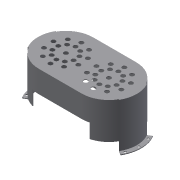
# Autodesk Inventor part: Gear Cover
Saved by Autodesk Inventor 2016 (Build 200138000, 138)
## iProperties
Created: 2012-10-11
Part Number: Gear Cover
Material: Generic
Document SubType Name: Sheet Metal
Designer: bruno.silveira
Density: 1 g/cm^3
Sheet Metal Rule: Default_mm
Flat Pattern Width: 75 cm
Flat Pattern Length: 33.7048 cm
Flat Pattern Area: 2527.86 cm^2
Sheet Metal Width: 750.000 mm
Sheet Metal Length: 337.048 mm
Sheet Metal Area: 252785.840 mm^2
Appearance: Default
Mass: 3205.56 g
Surface Area: 13697.7 cm^2
Volume: 3205.56 cm^3
Author: bruno.silveira
Autodesk Inventor part; units mm, degrees
ref_plane "YZ Plane" through (0, 0, 0) normal (1, 0, 0) x (0, 1, 0)
ref_plane "XZ Plane" through (0, 0, 0) normal (0, 1, 0) x (-1, 0, 0)
ref_plane "XY Plane" through (0, 0, 0) normal (0, 0, 1) x (1, 0, 0)
sketch "Sketch1" plane through (0, 0, 0) normal (0, 0, 1) x (1, 0, 0)
  circle A0 centre (0, 0) radius 190
  circle A1 centre (300, 0) radius 190
  line L0 (0, 190) -> (300, 190)
  line L1 (0, -190) -> (300, -190)
  dimension "d0" = 380
  dimension "d1" = 380
  dimension "d2" = 300
  measures "d0" diameter of A0
  measures "d1" diameter of A1
  measures "d2" distance of point (0, 0) A1.centre
extrude "Plate1" add sketch "Sketch1" along normal blind 4
sketch "Sketch2" plane through (0, 0, 0) normal (0, 0, -1) x (-1, 0, 0)
  arc A0 (-300, 190) -> (-300, -190) centre (-300, 0) ccw projected
  line L0 (0, -190) -> (-300, -190) projected
  arc A1 (0, -190) -> (0, 190) centre (0, 0) ccw projected
  line L1 (-300, 190) -> (0, 190) projected
  arc A2 (0, -186) -> (0, 186) centre (0, 0) ccw
  line L2 (0, -186) -> (-300, -186)
  arc A3 (-300, 186) -> (-300, -186) centre (-300, 0) ccw
  line L3 (-300, 186) -> (0, 186)
  dimension "d4" = 4
  constraints: 4 end point, 4 point on circle, 2 centre point, 3 other
  measures "d4" distance between parallel lines of L1 L3
extrude "Extrusion1" add sketch "Sketch2" along normal blind 250
sketch "Sketch3" plane through (0, 0, 4) normal (0, 0, 1) x (1, 0, 0)
  arc A0 (300, -190) -> (300, 190) centre (300, 0) ccw projected
  arc A1 (0, 190) -> (0, -190) centre (0, 0) ccw projected
  circle A2 centre (0, 0) radius 15
  circle A3 centre (300, 0) radius 15
  circle A4 centre (300, 0) radius 117.5
  circle A5 centre (408.5558, 44.9653) radius 15
  circle A6 centre (300, 0) radius 72.5
  circle A7 centre (366.9813, 27.7445) radius 15
  circle A8 centre (0, 0) radius 117.5
  circle A9 centre (0, 0) radius 72.5
  circle A10 centre (117.5, 0) radius 15
  circle A11 centre (72.5, 0) radius 15
  dimension "d29" = 235
  dimension "d30" = 145
  dimension "d7" = 30
  dimension "d8" = 30
  dimension "d11" = 235
  dimension "d12" = 30
  dimension "d13" = 145
  dimension "d14" = 30
  dimension "d31" = 30
  dimension "d32" = 30
  constraints: 8 centre point, 5 coincident, 2 horizontal alignment, 4 other
  measures "d7" diameter of A2
  measures "d8" diameter of A3
  measures "d11" diameter of A4
  measures "d12" diameter of A5
  measures "d13" diameter of A6
  measures "d14" diameter of A7
  measures "d31" diameter of A10
  measures "d32" diameter of A11
hole "Hole2" at (408.5558, 44.9653, 4) at (366.9813, 27.7445, 4) at (300, 0, 4) direction (0, 0, -1) diameter 30 depth 4 tip angle 118
pattern_circular "Circular Pattern2" count 10 over 360 about axis through (300, 0, 2) along (0, 0, 1) of "Hole2"
pattern_linear "Rectangular Pattern2" count 2 spacing 300 along (-1, 0, 0) of "Hole2", "Circular Pattern2"
sketch "Sketch4" plane through (0, -190, 4) normal (0, -1, 0) x (1, 0, 0)
  line L0 (0, -254) -> (0, 0) projected
  line L1 (0, -254) -> (300, -254) projected
  line L2 (-50, -154) -> (350, -154)
  line L3 (350, -154) -> (350, -254)
  line L4 (350, -254) -> (-50, -254)
  line L5 (-50, -254) -> (-50, -154)
  point P0 (0, -4)
  dimension "d49" = 400
  dimension "d50" = 50
  dimension "d51" = 100
  dimension "d52" = 0
  constraints: 8 end point, 2 parallel, 1 horizontal, 1 perpendicular
  measures "d49" distance of L3.end L4.end
  measures "d50" distance between parallel lines of L0 L5
  measures "d51" distance of L2.end L3.end
  measures "d52" distance between parallel lines of L1 L4
extrude "Cut1" cut sketch "Sketch4" against normal blind 10
sketch "Sketch5" plane through (0, 0, -250) normal (0, 0, -1) x (-1, 0, 0)
  line L0 (-300, 186) -> (0, 186) projected
  line L1 (-300, 190) -> (0, 190) projected
  line L2 (-350, -183.303) -> (-350, -180) projected
  line L3 (0, 190) -> (0, 186)
  line L4 (-300, 190) -> (-300, 186)
  constraints: 4 end point, 2 parallel
extrude "Extrusion2" add sketch "Sketch5" along normal blind 50
sketch "Sketch6" plane through (0, 186, -296) normal (0, 0, -1) x (-1, 0, 0)
  line L0 (-300, 0) -> (0, 0)
  line L1 (0, 0) -> (0, 40)
  line L2 (0, 40) -> (-300, 40)
  line L3 (-300, 40) -> (-300, 0)
  constraints: 6 end point, 1 horizontal, 1 perpendicular, 1 vertical
edge flange "Flange1" height 40 angle 90 thickness 4 bend radius 4 thickness toward (0, 0, -1) relief tear relief width 4 relief depth 2 edges at (150, 190, -300) wall of the first edge with corners at (300, 186, -296) (0, 186, -296) (0, 226, -296) (300, 226, -296)
bend "Bend1"
corner "Corner1"
sketch "Sketch7" plane through (0, 0, 4) normal (0, 0, 1) x (1, 0, 0)
  arc A0 (300, -190) -> (300, 190) centre (300, 0) ccw projected
  line L0 (0, 190) -> (300, 190) projected
  line L1 (300, -190) -> (0, -190) projected
  arc A1 (468.875, -97.5) -> (468.875, 97.5) centre (300, 0) ccw
  line L2 (464.5448, 95) -> (468.875, 97.5)
  line L3 (464.5448, -95) -> (468.875, -97.5)
  line L4 (150, 190) -> (150, -190)
  arc A2 (464.5448, -95) -> (464.5448, 95) centre (300, 0) ccw
  arc A3 (-168.875, 97.5) -> (-168.875, -97.5) centre (0, 0) ccw
  line L5 (-164.5448, 95) -> (-168.875, 97.5)
  line L6 (-164.5448, -95) -> (-168.875, -97.5)
  arc A4 (-164.5448, 95) -> (-164.5448, -95) centre (0, 0) ccw
  dimension "d67" = 5
  constraints: 12 end point, 8 point on circle, 6 symmetric about line, 4 centre point, 2 coincident, 2 midpoint, 2 other
  measures "d67" radial gap between concentric circles of A0 A1
extrude "Extrusion3" add sketch "Sketch7" against normal blind 310 contours A0 L2 A1 L3 | L5 A4 L6 A3
sketch "Sketch8" plane through (0, 0, -306) normal (0, 0, -1) x (-1, 0, 0)
  line L0 (-468.875, 97.5) -> (-464.5448, 95) projected
  arc A0 (-468.875, 97.5) -> (-468.875, -97.5) centre (-300, 0) ccw projected
  line L1 (-464.5448, -95) -> (-468.875, -97.5) projected
  arc A1 (-464.5448, 95) -> (-464.5448, -95) centre (-300, 0) ccw projected
  arc A2 (164.5448, -95) -> (164.5448, 95) centre (0, 0) ccw projected
  line L2 (168.875, -97.5) -> (164.5448, -95) projected
  arc A3 (168.875, -97.5) -> (168.875, 97.5) centre (0, 0) ccw projected
  line L3 (164.5448, 95) -> (168.875, 97.5) projected
  line L4 (164.5448, 95) -> (194.8557, 112.5)
  arc A4 (194.8557, -112.5) -> (194.8557, 112.5) centre (0, 0) ccw
  line L5 (164.5448, -95) -> (194.8557, -112.5)
  arc A5 (168.875, -97.5) -> (168.875, 97.5) centre (0, 0) ccw
  circle A6 centre (-47.085, -55.1294) radius 15 projected
  circle A7 centre (-76.3101, -89.3477) radius 15 projected
  circle A8 centre (37.8811, -61.8164) radius 15 projected
  circle A9 centre (61.3936, -100.1852) radius 15 projected
  circle A10 centre (70.4968, 16.9248) radius 15 projected
  circle A11 centre (114.2535, 27.4298) radius 15 projected
  circle A12 centre (5.6883, 72.2765) radius 15 projected
  circle A13 centre (9.2189, 117.1378) radius 15 projected
  circle A14 centre (-37.8811, 61.8164) radius 15 projected
  circle A15 centre (-61.3936, 100.1852) radius 15 projected
  circle A16 centre (76.3101, 89.3477) radius 15 projected
  circle A17 centre (47.085, 55.1294) radius 15 projected
  circle A18 centre (108.5558, -44.9653) radius 15 projected
  circle A19 centre (66.9813, -27.7445) radius 15 projected
  circle A20 centre (-9.2189, -117.1378) radius 15 projected
  circle A21 centre (-5.6883, -72.2765) radius 15 projected
  circle A22 centre (-114.2535, -27.4298) radius 15 projected
  circle A23 centre (-70.4968, -16.9248) radius 15 projected
  circle A24 centre (0, 0) radius 15 projected
  circle A25 centre (-66.9813, 27.7445) radius 15 projected
  circle A26 centre (-108.5558, 44.9653) radius 15 projected
  circle A27 centre (-347.085, -55.1294) radius 15 projected
  circle A28 centre (-376.3101, -89.3477) radius 15 projected
  circle A29 centre (-262.1189, -61.8164) radius 15 projected
  circle A30 centre (-238.6064, -100.1852) radius 15 projected
  circle A31 centre (-229.5032, 16.9248) radius 15 projected
  circle A32 centre (-185.7465, 27.4298) radius 15 projected
  circle A33 centre (-294.3117, 72.2765) radius 15 projected
  circle A34 centre (-290.7811, 117.1378) radius 15 projected
  circle A35 centre (-337.8811, 61.8164) radius 15 projected
  circle A36 centre (-361.3936, 100.1852) radius 15 projected
  circle A37 centre (-223.6899, 89.3477) radius 15 projected
  circle A38 centre (-252.915, 55.1294) radius 15 projected
  circle A39 centre (-191.4442, -44.9653) radius 15 projected
  circle A40 centre (-233.0187, -27.7445) radius 15 projected
  circle A41 centre (-309.2189, -117.1378) radius 15 projected
  circle A42 centre (-305.6883, -72.2765) radius 15 projected
  circle A43 centre (-414.2535, -27.4298) radius 15 projected
  circle A44 centre (-370.4968, -16.9248) radius 15 projected
  circle A45 centre (-300, 0) radius 15 projected
  circle A46 centre (-366.9813, 27.7445) radius 15 projected
  circle A47 centre (-408.5558, 44.9653) radius 15 projected
  line L6 (-300, -186) -> (0, -186) projected
  arc A48 (0, -186) -> (0, 186) centre (0, 0) ccw projected
  line L7 (0, 186) -> (-300, 186) projected
  arc A49 (-300, 186) -> (-300, -186) centre (-300, 0) ccw projected
  line L8 (-150, 186) -> (-150, -186)
  arc A50 (-468.875, 97.5) -> (-468.875, -97.5) centre (-300, 0) ccw
  line L9 (-468.875, 97.5) -> (-494.8557, 112.5)
  arc A51 (-494.8557, 112.5) -> (-494.8557, -112.5) centre (-300, 0) ccw
  line L10 (-468.875, -97.5) -> (-494.8557, -112.5)
  arc A52 (-468.875, 97.5) -> (-468.875, -97.5) centre (-300, 0) ccw
  dimension "d70" = 450
  constraints: 16 point on circle, 10 end point, 9 symmetric about line, 5 centre point, 4 coincident, 2 collinear, 2 midpoint, 2 point on line, 3 other
  measures "d70" diameter of A4
extrude "Extrusion4" add sketch "Sketch8" along normal blind 5 contours L0 A1 L1 A0 | A0 L10 A51 L9 | A2 L3 A3 L2 | A3 L4 A4 L5
sketch "Sketch9" plane through (0, 0, -306) normal (0, 0, 1) x (1, 0, 0)
  arc A0 (494.8557, -112.5) -> (494.8557, 112.5) centre (300, 0) ccw projected
  circle A1 centre (510, 0) radius 7.5
  circle A2 centre (300, 0) radius 210
  point P0 (0, 0)
  dimension "d74" = 420
  dimension "d73" = 15
  constraints: 1 centre point, 1 coincident, 1 horizontal alignment, 2 other
  measures "d73" diameter of A1
hole "Hole3" at (510, 0, -306) direction (0, 0, -1) diameter 15 end through all
pattern_circular "Circular Pattern3" count 3 over 45 about axis through (300, 0, 4) along (0, 0, 1) of "Hole3" both ways yes
sketch "Sketch10" plane through (0, 0, -306) normal (0, 0, 1) x (1, 0, 0)
  arc A0 (-194.8557, 112.5) -> (-194.8557, -112.5) centre (0, 0) ccw projected
  circle A1 centre (-210, 0) radius 7.5
  circle A2 centre (0, 0) radius 210
  dimension "d86" = 420
  dimension "d85" = 15
  constraints: 1 centre point, 1 coincident, 1 horizontal alignment, 2 other
  measures "d85" diameter of A1
hole "Hole4" at (-210, 0, -306) direction (0, 0, -1) diameter 15 end through all
pattern_circular "Circular Pattern4" count 3 over 45 about axis through (0, 0, 4) along (0, 0, 1) of "Hole4" both ways yes
sketch "Sketch11" plane through (0, 226, -296) normal (0, 0, 1) x (1, 0, 0)
  line L0 (0, 0) -> (0, -32) projected
  circle A0 centre (50, -16) radius 7.5
  point P0 (0, -226)
  dimension "d97" = 15
  dimension "d98" = 50
  constraints: 1 centre point
  measures "d97" diameter of A0
  measures "d98" distance from line of L0 A0.centre
hole "Hole5" at (50, 210, -296) direction (0, 0, -1) diameter 15 end through all
pattern_linear "Rectangular Pattern3" count 3 spacing 100 along (1, 0, 0) of "Hole5"
equation "\"d41\" = Thickness"
equation "\"d80\" = Thickness"
equation "\"d92\" = Thickness"
equation "\"d104\" = Thickness"
equation "\"d57\" = BendReliefWidth"
equation "\"d58\" = BendReliefDepth"
equation "\"d59\" = MinimumRemnant"
equation "\"d60\" = BendRadius"
equation "\"d63\" = BendRadius"
equation "\"d64\" = CornerReliefSize"
equation "\"d65\" = GapSize"
equation "\"d66\" = JacobiRadiusSize"
equation "\"BendRadius\" = Thickness"
equation "\"BendReliefWidth\" = Thickness"
equation "\"BendReliefDepth\" = 0.5 * Thickness"
equation "\"CornerReliefSize\" = 4 * Thickness"
equation "\"MinimumRemnant\" = 2 * Thickness"
equation "\"TransitionRadius\" = BendRadius"
equation "\"JacobiRadiusSize\" = BendRadius"
equation "\"GapSize\" = Thickness"
equation "\"d3\" = BendRadius"
equation "\"Thickness\" = 4"
body "Solid1"
